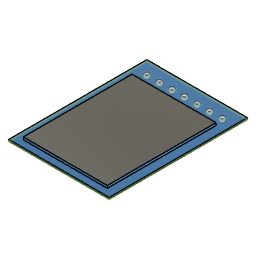
PERIMETRO_DISPLAY_TFT v3 (Autodesk Fusion 360 design; units mm, degrees)
Autodesk Fusion 360 part; units mm, degrees
sketch "Esboço1" plane through (0, 0, 0) normal (0, 0, 1) x (1, 0, 0)
  line L0 (-2.54, 2.54) -> (17.78, 2.54)
  line L1 (17.78, 2.54) -> (17.78, -25.4)
  line L2 (17.78, -25.4) -> (-2.54, -25.4)
  line L3 (-2.54, -25.4) -> (-2.54, 2.54)
  constraint horizontal L0
  constraint vertical L1
  constraint horizontal L2
  constraint vertical L3
extrude "Extrusão1" add sketch "Esboço1" along normal blind 0.3
sketch "Esboço2" plane through (0, 0, 0) normal (0, 0, 1) x (1, 0, 0)
  line L0 (-1, -2) -> (16, -2)
  line L1 (16, -2) -> (16, -24)
  line L2 (16, -24) -> (-1, -24)
  line L3 (-1, -24) -> (-1, -2)
  constraint horizontal L0
  constraint vertical L1
  constraint horizontal L2
  constraint vertical L3
extrude "Extrusão2" add sketch "Esboço2" along normal blind 0.8
sketch "Esboço3" plane through (0, 0, 0.3) normal (0, 0, 1) x (-1, 0, 0)
  line L0 (1, 24) -> (1, 2)
  line L1 (1, 2) -> (-16, 2)
  line L2 (-16, 2) -> (-16, 24)
  line L3 (-16, 24) -> (1, 24)
  line L4 (2.54, 25.4) -> (-17.78, 25.4)
  line L5 (-17.78, 25.4) -> (-17.78, -2.54)
  line L6 (-17.78, -2.54) -> (2.54, -2.54)
  line L7 (2.54, -2.54) -> (2.54, 25.4)
  circle A0 centre (0, 0) radius 0.25
  circle A1 centre (-2.5, 0) radius 0.25
  circle A2 through (-4.8305, 0.0007, -0.3) (-5.2055, 0.2172, -0.3) (-5.2055, -0.2158, -0.3)
  circle A3 centre (-7.62, 0.0108) radius 0.25
  circle A4 centre (-10.15, 0) radius 0.25
  circle A5 centre (-12.7077, 0.0204) radius 0.25
  circle A6 centre (-15.239, 0.0204) radius 0.25
  dimension "d5" = 0.5
  dimension "d6" = 0.5
  dimension "d7" = 0.5
  dimension "d8" = 0.5
  dimension "d9" = 0.5
  dimension "d10" = 0.5
  dimension "d11" = 0.5
  constraint coincident A0.centre origin
  measures "d5" diameter of A0
  measures "d6" diameter of A1
  measures "d8" diameter of A3
  measures "d9" diameter of A4
  measures "d10" diameter of A5
  measures "d11" diameter of A6
extrude "Extrusão3" cut sketch "Esboço3" against normal blind 0.05 contours A3 | A4 | A5 | A6
sketch "Esboço4" plane through (0, 0, 0.3) normal (0, 0, 1) x (-1, 0, 0)
  circle A0 centre (-12.7077, 0.0204) radius 0.25
  circle A1 centre (-10.15, 0) radius 0.25
  circle A2 centre (-15.239, 0.0204) radius 0.25
  circle A3 centre (-7.62, 0.0108) radius 0.25
  line L0 (1, 24) -> (1, 2)
  line L1 (1, 2) -> (-16, 2)
  line L2 (-16, 2) -> (-16, 24)
  line L3 (-16, 24) -> (1, 24)
  line L4 (2.54, 25.4) -> (-17.78, 25.4)
  line L5 (-17.78, 25.4) -> (-17.78, -2.54)
  line L6 (-17.78, -2.54) -> (2.54, -2.54)
  line L7 (2.54, -2.54) -> (2.54, 25.4)
  circle A4 centre (-5.0796, 0.0001) radius 0.25
  circle A5 centre (-2.54, 0) radius 0.25
  circle A6 centre (0, 0) radius 0.25
  dimension "d14" = 0.5
  dimension "d15" = 0.5
  dimension "d16" = 0.5
  constraint coincident A6.centre origin
  measures "d14" diameter of A4
  measures "d15" diameter of A5
  measures "d16" diameter of A6
extrude "Extrusão4" cut sketch "Esboço4" against normal blind 0.05 contours A4 | A5 | A6
sketch "Esboço5" plane through (0, 0, 0.3) normal (0, 0, 1) x (-1, 0, 0)
  circle A0 centre (-5.0796, 0.0001) radius 0.25
  circle A1 centre (-2.54, 0) radius 0.25
  circle A2 centre (0, 0) radius 0.25
  circle A3 centre (-12.7077, 0.0204) radius 0.25
  circle A4 centre (-10.15, 0) radius 0.25
  circle A5 centre (-15.239, 0.0204) radius 0.25
  circle A6 centre (-7.62, 0.0108) radius 0.25
  line L0 (1, 24) -> (1, 2)
  line L1 (1, 2) -> (-16, 2)
  line L2 (-16, 2) -> (-16, 24)
  line L3 (-16, 24) -> (1, 24)
  line L4 (2.54, 25.4) -> (-17.78, 25.4)
  line L5 (-17.78, 25.4) -> (-17.78, -2.54)
  line L6 (-17.78, -2.54) -> (2.54, -2.54)
  line L7 (2.54, -2.54) -> (2.54, 25.4)
  circle A7 centre (0, 0) radius 0.1
  circle A8 centre (-2.54, 0) radius 0.1
  circle A9 centre (-5.0796, 0.0001) radius 0.1
  circle A10 centre (-7.62, 0.0108) radius 0.1
  circle A11 centre (-10.15, 0) radius 0.1
  circle A12 centre (-12.7077, 0.0204) radius 0.1
  circle A13 centre (-15.239, 0.0204) radius 0.1
  dimension "d19" = 0.2
  dimension "d20" = 0.2
  dimension "d21" = 0.2
  dimension "d22" = 0.2
  dimension "d23" = 0.2
  dimension "d24" = 0.2
  dimension "d25" = 0.2
  constraint coincident A2.centre A7.centre
  constraint concentric A1 A8
  constraint concentric A0 A9
  constraint concentric A6 A10
  constraint concentric A4 A11
  constraint concentric A3 A12
  constraint concentric A5 A13
  measures "d19" diameter of A7
  measures "d20" diameter of A8
  measures "d21" diameter of A9
  measures "d22" diameter of A10
  measures "d23" diameter of A11
  measures "d24" diameter of A12
  measures "d25" diameter of A13
extrude "Extrusão5" cut sketch "Esboço5" against normal blind 2 contours A7 | A8 | A9 | A10 | A11 | A12 | A13
